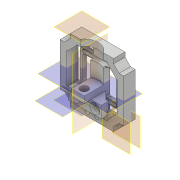
# Autodesk Inventor part: 20_Cube_Inser_Flexuremanipulator_zonly_translation_v3
Saved by Autodesk Inventor 2019.4 (Build 234330000, 330)
## iProperties
Created: 2019-07-01
Part Number: 20_Cube_Inser_Flexuremanipulator_zonly_translation_v3
Material: Generic
Document SubType Name: Modeling
Designer: diederichbenedict
Density: 1 g/cm^3
Appearance: Default
Author: diederichbenedict
Autodesk Inventor part; units mm, degrees
ref_plane "YZ Plane" through (0, 0, 0) normal (1, 0, 0) x (0, 1, 0)
ref_plane "XZ Plane" through (0, 0, 0) normal (0, 1, 0) x (-1, 0, 0)
ref_plane "Work Plane1" through (0, 0, 10) normal (0, 0, 1) x (1, 0, 0)
ref_plane "Work Plane4" through (0, 0, 13) normal (0, 0, 1) x (1, 0, 0)
sketch "Sketch5" plane through (0, 0, 13) normal (0, 0, 1) x (1, 0, 0)
  line L0 (-3.9299, 45.8299) -> (-37.9299, 45.8299) projected
  line L1 (-37.9299, 45.8299) -> (-37.9299, 42.2551) projected
  line L2 (-37.9299, 42.2551) -> (-42.2551, 37.9299) projected
  line L3 (-42.2551, 37.9299) -> (-45.8299, 37.9299) projected
  line L4 (-45.8299, 37.9299) -> (-45.8299, 3.9299) projected
  line L5 (-42.2551, 3.9299) -> (-45.8299, 3.9299) projected
  line L6 (-37.9299, -0.3953) -> (-42.2551, 3.9299) projected
  line L7 (-37.9299, -3.9701) -> (-37.9299, -0.3953) projected
  line L8 (-3.9713, -3.9701) -> (-37.9299, -3.9701) projected
  line L9 (-3.9713, -3.9701) -> (-3.9713, -0.4367) projected
  line L10 (-3.9713, -0.4367) -> (0.3953, 3.9299) projected
  line L11 (0.3953, 3.9299) -> (3.9701, 3.9299) projected
  line L12 (3.9701, 3.9299) -> (3.9701, 37.9299) projected
  line L13 (3.9701, 37.9299) -> (0.3953, 37.9299) projected
  line L14 (0.3953, 37.9299) -> (-3.9299, 42.2551) projected
  line L15 (-3.9299, 42.2551) -> (-3.9299, 45.8299) projected
  line L16 (-1.0299, 32.9299) -> (-1.0299, 8.9299)
  line L17 (-1.0299, 8.9299) -> (-1.6758, 8.9299)
  line L18 (-1.6758, 8.9299) -> (-8.9713, 1.6344)
  line L19 (-8.9713, 1.6344) -> (-8.9713, 1.0299)
  line L20 (-8.9713, 1.0299) -> (-32.9299, 1.0299)
  line L21 (-32.9299, 1.0299) -> (-32.9299, 1.6758)
  line L22 (-32.9299, 1.6758) -> (-40.184, 8.9299)
  line L23 (-40.184, 8.9299) -> (-40.8299, 8.9299)
  line L24 (-40.8299, 8.9299) -> (-40.8299, 32.9299)
  line L25 (-40.8299, 32.9299) -> (-40.184, 32.9299)
  line L26 (-40.184, 32.9299) -> (-32.9299, 40.184)
  line L27 (-32.9299, 40.184) -> (-32.9299, 40.8299)
  line L28 (-32.9299, 40.8299) -> (-8.9299, 40.8299)
  line L29 (-8.9299, 40.8299) -> (-8.9299, 40.184)
  line L30 (-8.9299, 40.184) -> (-1.6758, 32.9299)
  line L31 (-1.6758, 32.9299) -> (-1.0299, 32.9299)
  dimension "d46" = 5
  constraints: 32 end point, 15 other
  measures "d46" distance between parallel lines of L12 L16
extrude "Extrusion5" add sketch "Sketch5" along normal blind 6 and the other way blind 3
ref_plane "Work Plane5" through (0, 0, 21) normal (0, 0, 1) x (1, 0, 0)
sketch "Sketch7" plane through (0, 0, 10) normal (0, 0, 1) x (1, 0, 0)
  line L0 (-1.0299, 8.9299) -> (-1.6758, 8.9299) projected
  line L1 (-1.6758, 8.9299) -> (-8.9713, 1.6344) projected
  line L2 (-8.9713, 1.6344) -> (-8.9713, 1.0299) projected
  line L3 (-8.9713, 1.0299) -> (-32.9299, 1.0299) projected
  line L4 (-32.9299, 1.0299) -> (-32.9299, 1.6758) projected
  line L5 (-32.9299, 1.6758) -> (-40.184, 8.9299) projected
  line L6 (-40.184, 8.9299) -> (-40.8299, 8.9299) projected
  line L7 (-40.8299, 8.9299) -> (-40.8299, 32.9299) projected
  line L8 (-40.8299, 32.9299) -> (-40.184, 32.9299) projected
  line L9 (-40.184, 32.9299) -> (-32.9299, 40.184) projected
  line L10 (-32.9299, 40.184) -> (-32.9299, 40.8299) projected
  line L11 (-32.9299, 40.8299) -> (-8.9299, 40.8299) projected
  line L12 (-8.9299, 40.8299) -> (-8.9299, 40.184) projected
  line L13 (-8.9299, 40.184) -> (-1.6758, 32.9299) projected
  line L14 (-1.6758, 32.9299) -> (-1.0299, 32.9299) projected
  line L15 (-1.0299, 32.9299) -> (-1.0299, 8.9299) projected
  line L16 (-3.9299, 45.8299) -> (-37.9299, 45.8299) projected
  line L17 (-37.9299, 45.8299) -> (-37.9299, 42.2551) projected
  line L18 (-37.9299, 42.2551) -> (-42.2551, 37.9299) projected
  line L19 (-42.2551, 37.9299) -> (-45.8299, 37.9299) projected
  line L20 (-45.8299, 37.9299) -> (-45.8299, 3.9299) projected
  line L21 (-45.8299, 3.9299) -> (-42.2551, 3.9299) projected
  line L22 (-42.2551, 3.9299) -> (-37.9299, -0.3953) projected
  line L23 (-37.9299, -0.3953) -> (-37.9299, -3.9701) projected
  line L24 (-37.9299, -3.9701) -> (-3.9713, -3.9701) projected
  line L25 (-3.9713, -3.9701) -> (-3.9713, -0.4367) projected
  line L26 (-3.9713, -0.4367) -> (0.3953, 3.9299) projected
  line L27 (0.3953, 3.9299) -> (3.9701, 3.9299) projected
  line L28 (3.9701, 3.9299) -> (3.9701, 37.9299) projected
  line L29 (3.9701, 37.9299) -> (0.3953, 37.9299) projected
  line L30 (0.3953, 37.9299) -> (-3.9299, 42.2551) projected
  line L31 (-3.9299, 42.2551) -> (-3.9299, 45.8299) projected
  line L32 (-2.09, 9.9299) -> (-2.0299, 9.9299) projected
  line L33 (-2.0299, 9.9299) -> (-2.0299, 31.9299) projected
  line L34 (-2.0299, 31.9299) -> (-2.09, 31.9299) projected
  line L35 (-2.09, 31.9299) -> (-9.9299, 39.7698) projected
  line L36 (-9.9299, 39.7698) -> (-9.9299, 39.8299) projected
  line L37 (-9.9299, 39.8299) -> (-31.9299, 39.8299) projected
  line L38 (-31.9299, 39.8299) -> (-31.9299, 39.7698) projected
  line L39 (-31.9299, 39.7698) -> (-39.7698, 31.9299) projected
  line L40 (-39.7698, 31.9299) -> (-39.8299, 31.9299) projected
  line L41 (-39.8299, 31.9299) -> (-39.8299, 9.9299) projected
  line L42 (-39.8299, 9.9299) -> (-39.7698, 9.9299) projected
  line L43 (-39.7698, 9.9299) -> (-31.9299, 2.09) projected
  line L44 (-31.9299, 2.09) -> (-31.9299, 2.0299) projected
  line L45 (-31.9299, 2.0299) -> (-9.9713, 2.0299) projected
  line L46 (-9.9713, 2.0299) -> (-9.9713, 2.0486) projected
  line L47 (-9.9713, 2.0486) -> (-2.09, 9.9299) projected
  line L48 (-25.9299, 15.9299) -> (-20.9299, 15.9299)
  line L49 (-20.9299, 15.9299) -> (-20.9299, 31.9299)
  line L50 (-20.9299, 31.9299) -> (-25.9299, 31.9299)
  line L51 (-25.9299, 31.9299) -> (-25.9299, 15.9299)
  line L52 (-39.8299, 8.9299) -> (-39.8299, 32.9299) projected
  arc A0 (-39.8299, 30.9299) -> (-25.9299, 30.9299) centre (-32.8799, 31.9299) ccw construction
  line L53 (-25.9299, 30.9299) -> (-39.8299, 30.9299) construction
  line L54 (-25.9299, 30.9299) -> (-12.0299, 30.9299) construction
  line L55 (-39.8299, 31.9299) -> (-39.8299, 30.9299)
  line L56 (-25.9299, 30.9299) -> (-25.9299, 31.9299)
  line L57 (-25.9299, 15.9299) -> (-25.9299, 16.9299)
  arc A1 (-39.8299, 15.9299) -> (-25.9299, 15.9299) centre (-32.8799, 16.9299) ccw construction
  line L58 (-25.9299, 15.9299) -> (-39.8299, 15.9299) construction
  line L59 (-39.8299, 16.9299) -> (-39.8299, 15.9299)
  arc A2 (-39.8299, 16.9299) -> (-25.9299, 16.9299) centre (-32.8799, 16.9299) ccw construction
  circle A3 centre (-20.9299, 20.9299) radius 18.9
  line L60 (-25.9299, 15.9299) -> (-20.9299, 15.9299)
  line L61 (-20.9299, 15.9299) -> (-20.9299, 9.9299)
  line L62 (-20.9299, 9.9299) -> (-25.9299, 9.9299)
  line L63 (-25.9299, 9.9299) -> (-25.9299, 15.9299)
  line L64 (-20.9299, 31.9299) -> (-15.9299, 31.9299)
  line L65 (-15.9299, 31.9299) -> (-15.9299, 9.9299)
  line L66 (-15.9299, 9.9299) -> (-20.9299, 9.9299)
  line L67 (-20.9299, 9.9299) -> (-20.9299, 31.9299)
  point P0 (0, 0)
  point P1 (-39.7698, 16.9299)
  point P2 (-39.7698, 16.9299)
  dimension "d51" = 0
  dimension "d52" = 180
  dimension "d55" = 15
  dimension "d60" = 0
  dimension "d63" = 0
  dimension "d107" = 6
  dimension "d115" = 5
  dimension "d116" = 5
  dimension "d135" = 8.9
  dimension "d136" = 22
  constraints: 38 end point, 7 point on circle, 6 parallel, 4 centre point, 4 horizontal, 3 perpendicular, 2 collinear, 2 point on line, 2 tangent, 2 vertical, 1 concentric, 24 other
  measures "d52" angle of L53 L54
  measures "d60" distance from line of L57.start L48
  measures "d63" distance from line of A3.centre L49
  measures "d107" distance of L61.end L60.end
  measures "d115" distance between parallel lines of L49 L51
  measures "d116" distance of L65.end L61.end
  measures "d135" distance between parallel lines of L50 L11
  measures "d136" distance from line of L49.end L62
extrude "Extrusion6" add sketch "Sketch7" along normal up to surface (9 mm away) contours L51 L50 L49 L48 | L48 L61 L62 L63 | L49 L64 L65 L66 L61
sketch "Sketch10" plane through (0, 0, 19) normal (0, 0, 1) x (1, 0, 0)
  line L0 (-15.9299, 31.9299) -> (-15.9299, 9.9299) projected
  line L1 (-25.9299, 31.9299) -> (-15.9299, 31.9299) projected
  line L2 (-25.9299, 9.9299) -> (-25.9299, 31.9299) projected
  line L3 (-15.9299, 9.9299) -> (-25.9299, 9.9299) projected
  line L4 (-23.8799, 19.844) -> (-20.9799, 19.844) projected
  line L5 (-25.9299, 9.9299) -> (-25.9299, 31.9299) projected
  line L6 (-15.9299, 9.9299) -> (-15.9299, 31.9299) projected
  line L7 (-25.9299, 19.844) -> (-15.9299, 19.844)
  line L8 (-15.9299, 19.844) -> (-15.9299, 14.844)
  line L9 (-15.9299, 14.844) -> (-25.9299, 14.844)
  line L10 (-25.9299, 14.844) -> (-25.9299, 19.844)
  point P0 (0, 0)
  point P1 (-39.8299, 28.4889)
  point P2 (-2.0299, 28.4889)
  dimension "d140" = 5
  constraints: 8 end point, 2 parallel, 2 point on line, 1 horizontal, 1 perpendicular
  measures "d140" distance of L7.end L8.end
extrude "Extrusion9" add sketch "Sketch10" along normal blind 11 contours L0 L9 L2 L7 L4
ref_plane "Work Plane8" through (-37.9299, 45.8299, 10) normal (0, 1, 0) x (1, 0, 0)
ref_plane "Work Plane3" through (-27.93, 13.0477, 35) normal (0, -1, 0) x (1, 0, 0)
sketch "Sketch19" plane through (0, 0, 19) normal (0, 0, 1) x (1, 0, 0)
  line L0 (-23.3799, -3.9701) -> (-23.3799, 2.0299) projected
  line L1 (-18.4799, -3.9701) -> (-18.4799, 2.0299) projected
  circle A0 centre (-24.6083, -0.7296) radius 1.45
  circle A1 centre (-17.2627, -0.7296) radius 1.45
  point P0 (0, 0)
  dimension "d109" = 2.9
  dimension "d110" = 2.9
  constraints: 2 centre point
  measures "d109" diameter of A0
  measures "d110" diameter of A1
extrude "Extrusion17" cut sketch "Sketch19" against normal blind 7
sketch "Sketch20" plane through (0, 0, 10) normal (0, 0, -1) x (-1, 0, 0)
  line L0 (25.9299, 9.9299) -> (15.9299, 9.9299) projected
  line L1 (25.9299, 31.9299) -> (25.9299, 9.9299) projected
  line L2 (15.9299, 31.9299) -> (25.9299, 31.9299) projected
  line L3 (15.9299, 9.9299) -> (15.9299, 31.9299) projected
  line L4 (15.9299, 9.9299) -> (15.9299, 31.9299) projected
  line L5 (15.9299, 34.5094) -> (15.9299, 35.0094)
  line L6 (7.7745, 34.5094) -> (7.7745, 35.0094)
  line L7 (1.9699, 29.7049) -> (1.9699, 12.1049) projected
  line L8 (39.8899, 12.1049) -> (39.8899, 29.7049) projected
  line L9 (32.9299, 1.0299) -> (8.9713, 1.0299) projected
  line L10 (15.9299, 31.9299) -> (25.9299, 31.9299) projected
  line L11 (27.6381, 40.8299) -> (14.2217, 40.8299) projected
  line L12 (15.9299, 34.5094) -> (20.9299, 34.5094)
  line L13 (20.9299, 34.5094) -> (20.9299, 40.8299)
  line L14 (20.9299, 40.8299) -> (15.9299, 40.8299)
  line L15 (15.9299, 40.8299) -> (15.9299, 34.5094)
  line L16 (15.9299, 27.9299) -> (15.9299, 31.9299)
  line L17 (5.7745, 31.9299) -> (7.7745, 31.9299)
  line L18 (7.7745, 31.9299) -> (7.7745, 35.0094)
  line L19 (7.7745, 35.0094) -> (5.7745, 35.0094)
  line L20 (5.7745, 35.0094) -> (5.7745, 31.9299)
  line L21 (20.9299, 34.5094) -> (15.9299, 34.5094)
  line L22 (15.9299, 34.5094) -> (15.9299, 33.9799)
  line L23 (5.7745, 35.0094) -> (7.7745, 35.0094)
  line L24 (15.9299, 53.9299) -> (15.9299, 31.9299)
  line L25 (15.9299, 53.9299) -> (15.9299, 31.9299)
  line L26 (15.9299, 29.3504) -> (15.9299, 28.8504)
  line L27 (7.7745, 29.3504) -> (7.7745, 28.8504)
  line L28 (15.9299, 35.9299) -> (15.9299, 31.9299)
  line L29 (7.7745, 31.9299) -> (7.7745, 28.8504)
  line L30 (5.7745, 28.8504) -> (5.7745, 31.9299)
  line L31 (20.9299, 29.3504) -> (15.9299, 29.3504)
  line L32 (15.9299, 29.3504) -> (15.9299, 29.8799)
  line L33 (7.7745, 28.8504) -> (7.7745, 28.8504)
  line L34 (5.7745, 28.8504) -> (5.7745, 28.8504)
  line L35 (7.7745, 28.8504) -> (7.7745, 20.9299)
  line L36 (7.7745, 20.9299) -> (5.7745, 20.9299)
  line L37 (5.7745, 20.9299) -> (5.7745, 28.8504)
  line L38 (15.9299, 34.5094) -> (7.7745, 34.5094)
  line L39 (7.7745, 34.5094) -> (7.7745, 35.0094)
  line L40 (7.7745, 35.0094) -> (15.9299, 35.0094)
  line L41 (15.9299, 35.0094) -> (15.9299, 34.5094)
  line L42 (7.7745, 31.9299) -> (7.7745, 31.4299)
  line L43 (15.9299, 31.4299) -> (15.9299, 31.9299)
  line L44 (15.9299, 31.9299) -> (15.9299, 19.844) projected
  line L45 (7.7745, 31.9299) -> (15.9299, 31.9299)
  line L46 (15.9299, 31.9299) -> (15.9299, 31.4299)
  line L47 (15.9299, 31.4299) -> (7.7745, 31.4299)
  line L48 (7.7745, 31.4299) -> (7.7745, 31.9299)
  point P0 (0, 0)
  dimension "d1" = 0.5
  dimension "d151" = 0
  dimension "d152" = 0
  dimension "d162" = 0
  dimension "d163" = 2
  dimension "d164" = 0.5
  dimension "d165" = 0.5
  dimension "d166" = 0
  constraints: 76 end point, 11 symmetric about line, 10 parallel, 6 horizontal, 5 perpendicular, 2 point on line, 1 midpoint, 2 other
  measures "d1" distance of L5.end L5.start
  measures "d151" distance between parallel lines of L3 L15
  measures "d152" distance between parallel lines of L5 L22
  measures "d162" distance between parallel lines of L30 L37
  measures "d163" distance between parallel lines of L37 L35
  measures "d164" distance of L42.end L42.start
  measures "d165" distance of L45.end L46.end
  measures "d166" distance between parallel lines of L2 L45
extrude "Extrusion18" add sketch "Sketch20" against normal blind 3 contours L0 L3 L2 L1 | L3 L47 L29 L45 | L29 L27 L35 L36 L37 L30 L17 | L17 L20 L19 L6 L18 | L38 L6 L40 L5 | L5 L15 L11 L13 L12
ref_plane "Work Plane9" through (-20.9299, 3.9299, 19) normal (1, 0, 0) x (0, 0, -1)
ref_plane "Work Plane10" through (-37.9299, 20.9299, 19) normal (0, -1, 0) x (1, 0, 0)
mirror "Mirror2" about plane through (-20.9299, 3.9299, 19) normal (1, 0, 0) of "Extrusion18"
mirror "Mirror3" about plane through (-37.9299, 20.9299, 19) normal (0, -1, 0) of "Extrusion18", "Mirror2"
ref_plane "Work Plane11" through (-37.9299, -3.9701, 10) normal (0, -1, 0) x (1, 0, 0)
sketch "Sketch8" plane through (-37.9299, -3.9701, 10) normal (0, -1, 0) x (1, 0, 0)
  line L0 (12.756, 11) -> (21.244, 11) projected
  line L1 (12.756, 4) -> (21.244, 4) projected
  circle A0 centre (17, 5.6001) radius 2.45
  line L2 (21.244, 11) -> (21.244, 4) projected
  line L3 (12.756, 4) -> (12.756, 11) projected
  point P0 (37.9299, -10)
  dimension "d67" = 4.9
  constraints: 1 centre point
  measures "d67" diameter of A0
extrude "Extrusion7" cut sketch "Sketch8" against normal blind 7 contours A0 L1 | L1 A0
sketch "Sketch21" plane through (-37.9299, 45.8299, 19) normal (0, 1, 0) x (1, 0, 0)
  circle A0 centre (16.9, -6.047) radius 2.9 projected
  line L0 (12, 0) -> (22, 0) projected
  line L1 (12, 0) -> (12, -11) projected
  line L2 (22, -11) -> (12, -11) projected
  line L3 (22, 0) -> (22, -11) projected
  circle A1 centre (16.9, -6.047) radius 11
  point P0 (37.9299, 19)
  dimension "d137" = 22
  constraints: 1 centre point, 1 coincident
  measures "d137" diameter of A1
extrude "Extrusion19" cut sketch "Sketch21" against normal up to surface (25.986 mm away) contours A1
sketch "Sketch22" plane through (-25.9299, 19.844, 30) normal (0, 1, 0) x (1, 0, 0)
  circle A0 centre (5, 4.953) radius 0.7496 projected
  circle A1 centre (5, 4.953) radius 2.95
  point P0 (25.9299, 30)
  dimension "d141" = 5.9
  constraints: 1 centre point, 1 coincident
  measures "d141" diameter of A1
extrude "Extrusion20" cut sketch "Sketch22" against normal blind 10 contours A0 | A1
sketch "Sketch23" plane through (-15.9299, 14.844, 30) normal (1, 0, 0) x (0, 0, -1)
  line L0 (4.753, 12.51) -> (4.753, 13)
  line L1 (5.7026, 0.75) -> (5.7026, 11)
  spline S0 degree 2 poles (6.6273, 8.464) (4.953, 9.7248) (3.2787, 8.464) knots 0.427493 0.427493 0.427493 1.087645 1.087645 1.087645 weights 1.448918 1.6593 1.448918 projected
  line L2 (3.2787, 8.464) -> (3.2787, 5) projected
  line L3 (3.2787, 5) -> (6.6273, 5) projected
  line L4 (6.6273, 5) -> (6.6273, 8.464) projected
  line L5 (4.2034, 0.75) -> (4.2034, 11)
  line L6 (11, 0) -> (0, 0) projected
  line L7 (11, 0) -> (11, 5) projected
  line L8 (11, 0) -> (5.3026, 0)
  line L9 (5.3026, 0) -> (5.3026, -4.914)
  line L10 (5.3026, -4.914) -> (11, -4.914)
  line L11 (11, -4.914) -> (11, 0)
  line L12 (11, -4.914) -> (5.3026, -9.3006)
  line L13 (5.3026, -9.3006) -> (5.3026, -4.914)
  line L14 (5.3026, -9.3006) -> (9.8399, -9.3006)
  line L15 (9.8399, -9.3006) -> (11, -4.914)
  point P0 (30, -14.844)
  point P1 (11, -0.914)
  dimension "d144" = 0.4
  constraints: 22 end point, 3 vertical, 2 horizontal, 2 parallel, 1 collinear, 1 perpendicular, 6 other
  measures "d144" distance between parallel lines of L9 L1
extrude "Extrusion21" add sketch "Sketch23" along normal blind 8 and the other way blind 18 contours L11 L10 L9 L6 | L12 L13 L10 | L15 L14 L12
sketch "Sketch24" plane through (-33.9299, 5.5434, 24.6974) normal (0, 0, 1) x (-1, 0, 0)
  line L0 (-26, 0) -> (0, 0) projected
  line L1 (0, 0) -> (0, -9.3006) projected
  line L2 (-15.9292, -9.3006) -> (-10.0708, -9.3006) projected
  circle A0 centre (-5, -4.6503) radius 3.95
  line L3 (-26, -9.3006) -> (-26, 0) projected
  line L4 (-26, -9.3006) -> (-18, -9.3006) projected
  line L5 (-15.9292, -9.3006) -> (-18, -9.3006) projected
  line L6 (-8, -9.3006) -> (-10.0708, -9.3006) projected
  line L7 (-8, -9.3006) -> (0, -9.3006) projected
  circle A1 centre (-21, -4.6503) radius 3.95
  point P0 (-33.9299, 5.5434)
  dimension "d147" = 7.9
  dimension "d170" = 5
  dimension "d171" = 7.9
  dimension "d172" = 5
  constraints: 2 centre point
  measures "d147" diameter of A0
  measures "d170" distance from line of L1 A0.centre
  measures "d171" diameter of A1
  measures "d172" distance from line of A1.centre L3
extrude "Extrusion22" cut sketch "Sketch24" against normal blind 4 contours A0 | A1
fillet "Fillet3" radius 1 20 edges at (-34.0854, 34.5094, 11.5) (-34.0854, 31.9299, 11.5) (-7.7745, 31.9299, 11.5) (-7.7745, 34.5094, 11.5) (-7.7745, 31.4299, 11.5) (-15.9299, 31.4299, 11.5) (-25.9299, 31.4299, 11.5) (-34.0854, 31.4299, 11.5) (-5.7745, 35.0094, 11.5) (-36.0854, 35.0094, 11.5) (-34.0854, 10.4299, 11.5) (-34.0854, 7.3504, 11.5) (-15.9299, 10.4299, 11.5) (-5.7745, 6.8504, 11.5) (-7.7745, 10.4299, 11.5) (-7.7745, 7.3504, 11.5) (-36.0854, 6.8504, 11.5) (-25.9299, 10.4299, 11.5) (-34.0854, 9.9299, 11.5) (-7.7745, 9.9299, 11.5)
chamfer "Chamfer3" distance 6 angle 45 2 edges at (-25.9299, 12.387, 19) (-15.9299, 12.387, 19)
body "Solid1"
